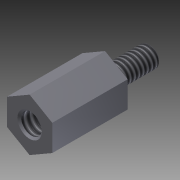
# Autodesk Inventor part: 219-1048
Saved by Autodesk Inventor 2011 (Build 150239000, 239)
## iProperties
Category: Control Systems
Company: Autodesk Inc.
Created: 2008-12-10
Part Number: 219-1048
Document SubType Name: Modeling
Designer: Autodesk Inc.
Density: 7.86 g/cm^3
Material: Steel, Mild
Catalog Web Link: http://www.alliedelec.com/Images/Products/Datasheets/BM/RAF_ELECTRONIC_HARDWARE/RAF-ELECTRONIC-HARDWARE_ENCLOSURE-AND-COOLING_2191006.PDF
Description: Standoff
Vendor: Allied Electronics
Mass: 1.16769 g
Surface Area: 2.45928 cm^2
Volume: 0.148561 cm^3
Author: Autodesk Inc.
Autodesk Inventor part; units mm, degrees
ref_plane "YZ Plane" through (0, 0, 0) normal (1, 0, 0) x (0, 1, 0)
ref_plane "XZ Plane" through (0, 0, 0) normal (0, 1, 0) x (-1, 0, 0)
sketch "Sketch2" plane through (0, 0, 0) normal (0, 0, 1) x (1, 0, 0)
  line L0 (2.3813, 1.3748) -> (2.3812, -1.3748)
  line L1 (2.3812, -1.3748) -> (0, -2.7496)
  line L2 (0, -2.7496) -> (-2.3812, -1.3748)
  line L3 (-2.3812, 1.3748) -> (-2.3812, -1.3748)
  line L4 (-2.3812, 1.3748) -> (0, 2.7496)
  line L5 (0, 2.7496) -> (2.3813, 1.3748)
  circle A0 centre (0, 0) radius 2.7496 construction
  line L6 (0, 25.4) -> (0, -25.4) construction
  dimension "d3" = 4.7625
  constraints: 14 end point, 6 point on circle, 3 equal length, 2 parallel, 2 vertical, 1 centre point, 1 point on line, 1 other
  measures "d3" distance between parallel lines of L1 L4
extrude "Hexagon1" add sketch "Sketch2" against normal blind 7.9375
sketch "Sketch3" plane through (0, 0, -7.9375) normal (0, 0, -1) x (-1, 0, 0)
  circle A0 centre (0, 0) radius 1.0795
  dimension "d11" = 2.159
  constraints: 1 centre point
  measures "d11" diameter of A0
sketch "Sketch4" plane through (0, 0, 0) normal (0, 0, 1) x (1, 0, 0)
  point P0 (0, 0)
hole "Hole1" at (0, 0, 0) direction (0, 0, -1) diameter 2.159 depth 6.35 tip angle 118
extrude "Extrusion2" add sketch "Sketch3" along normal blind 4.7625
chamfer "Chamfer1" distance 0.1984 angle 45 1 edges at (1.0795, 0, -12.7)
chamfer "Chamfer2" distance 0.1984 angle 45 1 edges at (0, 1.0795, 0)
thread "Thread1" size "2-56 UNC" class "2A" standard "ANSI Unified Screw Threads" full length
ref_plane "Work Plane1" through (0, 0, -12.6008) normal (0.866, -0.5, 0) x (0, 0, 1)
sketch "Sketch5" plane through (0, 0, -12.6008) normal (0.866, -0.5, 0) x (0, 0, 1)
  line L0 (4.6633, 0) -> (4.6633, -2.3812) projected
  line L1 (4.6633, -1.0795) -> (0.0992, -1.0795) projected
  line L2 (4.6633, -1.0795) -> (4.3763, -1.0795)
  line L3 (4.3763, -1.0795) -> (4.3763, -0.8769)
  line L4 (4.3763, -0.8769) -> (4.6633, -0.8769)
  line L5 (4.6633, -0.8769) -> (4.6633, -1.0795)
  line L6 (-2.6392, 0) -> (15.1408, 0) projected
  constraints: 8 end point, 2 parallel, 1 horizontal, 1 perpendicular
revolve "Revolution1" cut sketch "Sketch5" angle 360 about axis through (0, 0, -10) along (0, 0, 1)
chamfer "Chamfer3" distance 0.1984 angle 45 1 edges at (1.0795, 0, -8.2244)
body "Solid1"
